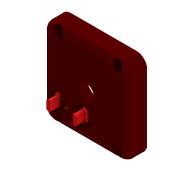
# Autodesk Inventor part: gearbox v2
Saved by Autodesk Inventor 2020.3 (Build 243373000, 373)
## iProperties
Created: 2020-05-25
Part Number: gearbox v2
Material: Generic
Document SubType Name: Modeling
Designer: stefa
Density: 1 g/cm^3
Appearance: Smooth - Red
Author: stefa
Autodesk Inventor part; units mm, degrees
ref_plane "YZ Plane" through (0, 0, 0) normal (1, 0, 0) x (0, 1, 0)
ref_plane "XZ Plane" through (0, 0, 0) normal (0, 1, 0) x (-1, 0, 0)
ref_plane "XY Plane" through (0, 0, 0) normal (0, 0, 1) x (1, 0, 0)
sketch "Sketch1" plane through (0, 0, 0) normal (0, 0, 1) x (1, 0, 0)
  line L0 (-25, -25) -> (25, -25)
  line L1 (25, -25) -> (25, 25)
  line L2 (25, 25) -> (-25, 25)
  line L3 (-25, 25) -> (-25, -25)
  line L4 (-25, -25) -> (25, 25) construction
  line L5 (25, -25) -> (-25, 25) construction
  line L6 (-15, 15) -> (15, 15)
  line L7 (15, 15) -> (15, -15)
  line L8 (15, -15) -> (-15, -15)
  line L9 (-15, -15) -> (-15, 15)
  circle A0 centre (0, 0) radius 11
  circle A1 centre (0, 0) radius 4.25
  circle A2 centre (-17, 21) radius 2
  circle A3 centre (17, 21) radius 2
  circle A4 centre (-17, -21) radius 2
  circle A5 centre (17, -21) radius 2
  dimension "d0" = 50
  dimension "d1" = 50
  dimension "d2" = 10
  dimension "d3" = 22
  dimension "d4" = 8.5
  dimension "d19" = 4
  dimension "d20" = 4
  dimension "d23" = 34
  dimension "d26" = 42
  dimension "d32" = 8
  constraints: 20 end point, 6 centre point, 4 parallel, 2 coincident, 2 horizontal, 2 midpoint, 2 perpendicular, 1 vertical, 9 other
  measures "d0" distance of L2.end L1.end
  measures "d1" distance of L1.end L0.end
  measures "d2" distance between parallel lines of L2 L6
  measures "d3" diameter of A0
  measures "d4" diameter of A1
  measures "d19" diameter of A2
  measures "d20" distance from line of L2 A2.centre
  measures "d23" distance of A2.centre A3.centre
  measures "d26" distance of A2.centre A4.centre
  measures "d32" distance from line of L3 A2.centre
extrude "Extrusion1" add sketch "Sketch1" along normal blind 10 contours L3 L2 L1 L0 | L6 L7 L8 L9 | A0 | A1 | A2 | A3 | A4 | A5
extrude "Extrusion3" cut sketch "Sketch1" along normal blind 9 contours A0
extrude "Extrusion4" cut sketch "Sketch1" along normal through all contours A2 | A3 | A4 | A5
extrude "Extrusion7" cut sketch "Sketch1" along normal through all contours A1
fillet "Fillet1" radius 6 4 edges at (-25, 25, 5) (-25, -25, 5) (25, 25, 5) (25, -25, 5)
sketch "Sketch4" plane through (0, 0, 10) normal (0, 0, 1) x (1, 0, 0)
  circle A0 centre (0, 0) radius 11 projected
  arc A1 (19, -25) -> (25, -19) centre (19, -19) ccw projected
  line L0 (25, -19) -> (25, 19) projected
  arc A2 (25, 19) -> (19, 25) centre (19, 19) ccw projected
  line L1 (19, 25) -> (-19, 25) projected
  arc A3 (-19, 25) -> (-25, 19) centre (-19, 19) ccw projected
  line L2 (-25, 19) -> (-25, -19) projected
  arc A4 (-25, -19) -> (-19, -25) centre (-19, -19) ccw projected
  line L3 (-19, -25) -> (19, -25) projected
  circle A5 centre (17, -21) radius 2 projected
  circle A6 centre (-17, -21) radius 2 projected
  circle A7 centre (17, 21) radius 2 projected
  circle A8 centre (-17, 21) radius 2 projected
  circle A9 centre (17, -21) radius 3.55
  circle A10 centre (-17, -21) radius 2 projected
  circle A11 centre (-17, -21) radius 3.55
  circle A12 centre (-17, 21) radius 3.55
  circle A13 centre (17, 21) radius 3.55
  dimension "d46" = 7.1
  constraints: 4 centre point, 4 coincident, 3 equal radius
  measures "d46" diameter of A9
extrude "Extrusion9" cut sketch "Sketch4" against normal blind 4 contours A6 | A9 | A11 | A12 | A13
fillet "Fillet3" radius 3.5 8 edges at (-23.2426, -23.2426, 10) (0, -25, 10) (23.2426, -23.2426, 10) (25, 0, 10) (23.2426, 23.2426, 10) (0, 25, 10) (-23.2426, 23.2426, 10) (-25, 0, 10)
sketch "Sketch5" plane through (0, 0, 10) normal (0, 0, 1) x (1, 0, 0)
  arc A0 (-12.6793, -15.3707) -> (-12.6086, -15.4) centre (-12.6086, -15.3) ccw projected
  line L0 (-12.6086, -15.4) -> (-11.0914, -15.4) projected
  arc A1 (-11.0914, -15.4) -> (-11.0207, -15.3707) centre (-11.0914, -15.3) ccw projected
  line L1 (-11.0207, -15.3707) -> (-10.6793, -15.0293) projected
  arc A2 (-10.6086, -15) -> (-10.6793, -15.0293) centre (-10.6086, -15.1) ccw projected
  line L2 (-10.6086, -15) -> (-6.4914, -15) projected
  arc A3 (-6.4207, -15.0293) -> (-6.4914, -15) centre (-6.4914, -15.1) ccw projected
  line L3 (-6.4207, -15.0293) -> (-6.0793, -15.3707) projected
  arc A4 (-6.0793, -15.3707) -> (-6.0086, -15.4) centre (-6.0086, -15.3) ccw projected
  line L4 (-6.0086, -15.4) -> (-4.6914, -15.4) projected
  arc A5 (-4.6914, -15.4) -> (-4.6207, -15.3707) centre (-4.6914, -15.3) ccw projected
  line L5 (-4.6207, -15.3707) -> (-4.2793, -15.0293) projected
  arc A6 (-4.2086, -15) -> (-4.2793, -15.0293) centre (-4.2086, -15.1) ccw projected
  line L6 (-4.2086, -15) -> (-2.4, -15) projected
  arc A7 (-2.4, -15) -> (-2.3, -14.9) centre (-2.4, -14.9) ccw projected
  line L7 (-2.3, -14.9) -> (-2.3, -12.6) projected
  line L8 (-2.3, -12.6) -> (-6.45, -12.6) projected
  arc A8 (-6.45, -12.6) -> (-6.95, -13.1) centre (-6.45, -13.1) ccw projected
  line L9 (-6.95, -13.1) -> (-6.95, -14.6) projected
  line L10 (-6.95, -14.6) -> (-10.35, -14.6) projected
  line L11 (-10.35, -14.6) -> (-10.35, -13.1) projected
  arc A9 (-10.35, -13.1) -> (-10.85, -12.6) centre (-10.85, -13.1) ccw projected
  line L12 (-10.85, -12.6) -> (-15, -12.6) projected
  line L13 (-15, -12.6) -> (-15, -14.9) projected
  arc A10 (-15, -14.9) -> (-14.9, -15) centre (-14.9, -14.9) ccw projected
  line L14 (-14.9, -15) -> (-13.0914, -15) projected
  arc A11 (-13.0207, -15.0293) -> (-13.0914, -15) centre (-13.0914, -15.1) ccw projected
  line L15 (-13.0207, -15.0293) -> (-12.6793, -15.3707) projected
  circle A12 centre (-5.35, -14) radius 1 projected
  arc A13 (-11.95, -13) -> (-11.95, -15) centre (-11.95, -14) ccw projected
  line L16 (-11.95, -13) -> (-11.75, -13) projected
  arc A14 (-11.75, -15) -> (-11.75, -13) centre (-11.75, -14) ccw projected
  line L17 (-11.75, -15) -> (-11.95, -15) projected
  line L18 (-15, -12.59) -> (-15, -9) projected
  line L19 (-2.3, -9) -> (-2.3, -12.59) projected
  line L20 (-14.9, -8.9) -> (-2.4, -8.9) projected
  line L21 (-11.75, -13.1) -> (-11.95, -13.1)
  arc A15 (-11.95, -13.1) -> (-11.95, -14.9) centre (-11.95, -14) ccw
  line L22 (-11.95, -14.9) -> (-11.75, -14.9)
  arc A16 (-11.75, -14.9) -> (-11.75, -13.1) centre (-11.75, -14) ccw
  circle A17 centre (-5.35, -14) radius 0.9
  line L23 (-4.6914, -15.6) -> (-6.0086, -15.6)
  arc A18 (-6.2207, -15.5121) -> (-6.0086, -15.6) centre (-6.0086, -15.3) ccw
  line L24 (-6.2207, -15.5121) -> (-6.5328, -15.2)
  line L25 (-6.5328, -15.2) -> (-10.5672, -15.2)
  line L26 (-10.5672, -15.2) -> (-10.8793, -15.5121)
  arc A19 (-11.0914, -15.6) -> (-10.8793, -15.5121) centre (-11.0914, -15.3) ccw
  line L27 (-11.0914, -15.6) -> (-12.6086, -15.6)
  arc A20 (-12.8207, -15.5121) -> (-12.6086, -15.6) centre (-12.6086, -15.3) ccw
  line L28 (-12.8207, -15.5121) -> (-13.1328, -15.2)
  line L29 (-13.1328, -15.2) -> (-14.9, -15.2)
  arc A21 (-15.2, -14.9) -> (-14.9, -15.2) centre (-14.9, -14.9) ccw
  line L30 (-15.2, -14.9) -> (-15.2, -12.4)
  line L31 (-15.2, -12.4) -> (-15, -12.4)
  line L32 (-2.3, -12.4) -> (-2.1, -12.4)
  line L33 (-2.1, -12.4) -> (-2.1, -14.9)
  arc A22 (-2.4, -15.2) -> (-2.1, -14.9) centre (-2.4, -14.9) ccw
  line L34 (-2.4, -15.2) -> (-4.1672, -15.2)
  line L35 (-4.1672, -15.2) -> (-4.4793, -15.5121)
  arc A23 (-4.6914, -15.6) -> (-4.4793, -15.5121) centre (-4.6914, -15.3) ccw
  line L36 (-12.6086, -15.6) -> (-11.1086, -15.6)
  line L37 (-11.1086, -15.6) -> (-11.1086, -16.6)
  line L38 (-11.1086, -16.6) -> (-12.6086, -16.6)
  line L39 (-12.6086, -16.6) -> (-12.6086, -15.6)
  line L40 (-8.55, -18.9088) -> (-8.55, -9.3296) construction
  line L41 (-15.2, -9.1) -> (-17.2, -9.1)
  line L42 (-17.2, -9.1) -> (-17.2, -14.6)
  line L43 (-17.2, -14.6) -> (-15.2, -14.6)
  line L44 (-15.2, -14.6) -> (-15.2, -9.1)
  line L45 (-4.4914, -15.6) -> (-5.9914, -15.6)
  line L46 (-5.9914, -15.6) -> (-5.9914, -16.6)
  line L47 (-5.9914, -16.6) -> (-4.4914, -16.6)
  line L48 (-4.4914, -16.6) -> (-4.4914, -15.6)
  line L49 (-1.9, -9.1) -> (0.1, -9.1)
  line L50 (0.1, -9.1) -> (0.1, -14.6)
  line L51 (0.1, -14.6) -> (-1.9, -14.6)
  line L52 (-1.9, -14.6) -> (-1.9, -9.1)
  line L53 (-25, 19) -> (-25, -19) projected
  arc A24 (-21.5, -19) -> (-20.5498, -20.9617) centre (-19, -19) ccw projected
  arc A25 (-13.4854, -21.5) -> (-20.5498, -20.9617) centre (-17, -21) ccw projected
  line L54 (13.4854, -21.5) -> (-13.4854, -21.5) projected
  arc A26 (20.5498, -20.9617) -> (13.4854, -21.5) centre (17, -21) ccw projected
  arc A27 (20.5498, -20.9617) -> (21.5, -19) centre (19, -19) ccw projected
  line L55 (21.5, 19) -> (21.5, -19) projected
  arc A28 (21.5, 19) -> (20.5498, 20.9617) centre (19, 19) ccw projected
  arc A29 (13.4854, 21.5) -> (20.5498, 20.9617) centre (17, 21) ccw projected
  line L56 (-13.4854, 21.5) -> (13.4854, 21.5) projected
  arc A30 (-20.5498, 20.9617) -> (-13.4854, 21.5) centre (-17, 21) ccw projected
  arc A31 (-20.5498, 20.9617) -> (-21.5, 19) centre (-19, 19) ccw projected
  line L57 (-21.5, -19) -> (-21.5, 19) projected
  circle A32 centre (0, 0) radius 4.25 projected
  circle A33 centre (-5.35, -14) radius 0.9
  arc A34 (-11.75, -14.9) -> (-11.75, -13.1) centre (-11.75, -14) ccw
  arc A35 (-11.95, -13.1) -> (-11.95, -14.9) centre (-11.95, -14) ccw
  line L58 (-11.95, -13.1) -> (-11.75, -13.1)
  line L59 (-11.95, -14.9) -> (-11.75, -14.9)
  point P0 (-15.2, -13.65)
  dimension "d12" = 0
  dimension "d50" = 0.1
  dimension "d51" = 0.1
  dimension "d52" = 0.2
  dimension "d53" = 0.2
  dimension "d54" = 0.2
  dimension "d55" = 0.2
  dimension "d56" = 1.5
  dimension "d57" = 1
  dimension "d58" = 2
  dimension "d59" = 5.5
  dimension "d60" = 0.6
  dimension "d61" = 16.45
  constraints: 68 end point, 20 point on circle, 12 centre point, 8 symmetric about line, 5 parallel, 3 coincident, 3 concentric, 3 horizontal, 3 point on line, 3 tangent, 2 perpendicular, 1 midpoint, 1 vertical, 18 other
  measures "d50" radial gap between concentric circles of A14 A16
  measures "d51" radial gap between concentric circles of A12 A17
  measures "d52" distance between parallel lines of L4 L23
  measures "d53" distance between parallel lines of L7 L33
  measures "d54" distance between parallel lines of L32 L8
  measures "d55" distance between parallel lines of L12 L31
  measures "d56" distance of L37.end L38.end
  measures "d57" distance of L36.end L37.end
  measures "d58" distance between parallel lines of L44 L42
  measures "d59" distance of L41.end L42.end
  measures "d60" distance between parallel lines of L29 L43
  measures "d61" distance between parallel lines of L53 L40
extrude "Extrusion10" add sketch "Sketch5" along normal blind 6 contours L43 L42 L41 L44 L30 | L49 L50 L51 L52
sketch "Sketch6" plane through (0, 0, 10) normal (0, 0, 1) x (1, 0, 0)
  point P0 (0, 0)
  point P1 (-5.3246, -13.9891)
  point P2 (-11.8716, -14.0197)
  point P3 (-11.7716, -13.9768)
  point P4 (-11.8836, -14.0009)
hole "Hole1" at (-5.3246, -13.9891, 10) at (-11.8836, -14.0009, 10) direction (0, 0, -1) diameter 1.567 depth 6.3 tip angle 118 thread size "M2x0.4" class "6H" standard "ISO Metric profile"
fillet "Fillet4" radius 1 10 edges at (-16.2, -14.6, 10) (-17.2, -11.85, 10) (-0.9, -14.6, 10) (0.1, -11.85, 10) (-0.9, -9.1, 10) (0.1, -9.1, 13) (0.1, -14.6, 13) (-17.2, -14.6, 13) (-17.2, -9.1, 13) (-16.2, -9.1, 10)
equation "\"d23\" = d1 - 2 * d32"
equation "\"d26\" = d0 - 2 * d20"
body "Solid1"
